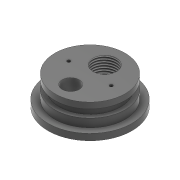
# Autodesk Inventor part: Pieza_sonar
Saved by Autodesk Inventor 2022.3 (Build 263350000, 350)
## iProperties
Created: 2023-07-17
Part Number: Pieza_sonar
Material: Genérico
Document SubType Name: Modeling
Designer: Usuario
Density: 1 g/cm^3
Appearance: Valor por defecto
Author: Usuario
Autodesk Inventor part; units mm, degrees
ref_plane "YZ Plane" through (0, 0, 0) normal (1, 0, 0) x (0, 1, 0)
ref_plane "XZ Plane" through (0, 0, 0) normal (0, 1, 0) x (-1, 0, 0)
sketch "Boceto1" plane through (0, 0, 0) normal (0, 1, 0) x (-1, 0, 0)
  circle A0 centre (0, 0) radius 26
  dimension "d0" = 52
  constraints: 1 centre point, 1 coincident
  measures "d0" diameter of A0
extrude "Extrusión1" add sketch "Boceto1" along normal blind 4
sketch "Boceto2" plane through (0, 4, 0) normal (0, 1, 0) x (1, 0, 0)
  circle A0 centre (0, 0) radius 21.775
  dimension "d3" = 43.55
  constraints: 1 centre point, 1 coincident
  measures "d3" diameter of A0
extrude "Extrusión2" add sketch "Boceto2" along normal blind 13.8
ref_plane "Plano de trabajo1" through (0, 14.2, 0) normal (0, 1, 0) x (1, 0, 0)
sketch "Boceto6" plane through (0, 14.2, 0) normal (0, 1, 0) x (1, 0, 0)
  circle A0 centre (0, 0) radius 21.775
  circle A1 centre (0, 0) radius 18.925
  dimension "d18" = 37.85
  constraints: 2 centre point, 2 coincident
  measures "d18" diameter of A1
extrude "Extrusión6" cut sketch "Boceto6" against normal blind 5
sketch "Boceto7" plane through (0, 0, 0) normal (0, -1, 0) x (1, 0, 0)
  circle A0 centre (0, 0) radius 18.925 projected
  circle A1 centre (0, 0) radius 21.775 projected
  circle A2 centre (0, 0) radius 26 projected
  line L0 (0, 26) -> (0, 20.5)
  line L1 (0, 20.5) -> (0, 3.45)
  arc A3 (8.0792, 17.1138) -> (4.3595, 20.5) centre (0, 11.975) ccw
  line L2 (0, 3.45) -> (4.3595, 3.45)
  line L3 (0, 3.45) -> (-4.3595, 3.45)
  line L4 (0, 20.5) -> (4.3595, 20.5)
  line L5 (0, 20.5) -> (-4.3595, 20.5)
  arc A4 (4.3595, 3.45) -> (8.0792, 17.1138) centre (0, 11.975) ccw
  arc A5 (-4.3595, 3.45) -> (4.3595, 3.45) centre (0, 11.975) ccw
  arc A6 (4.3595, 20.5) -> (-4.3595, 20.5) centre (0, 11.975) ccw
  arc A7 (-4.3595, 20.5) -> (-4.3595, 3.45) centre (0, 11.975) ccw
  dimension "d21" = 5.5
  dimension "d22" = 17.05
  dimension "d23" = 19.15
  constraints: 13 point on circle, 12 end point, 5 centre point, 2 point on line, 2 vertical, 1 horizontal, 1 midpoint, 1 parallel, 1 vertical alignment, 3 other
  measures "d21" distance of L0.start L0.end
  measures "d22" distance of L0.end L1.end
  measures "d23" diameter of A3
extrude "Extrusión7" cut sketch "Boceto7" against normal blind 4.45 contours A4 L2 L1 A0 | A0 L1 L4 A3 | A7 L5 L1 A0 | A0 L1 L3 A7
sketch "Boceto8" plane through (0, 4.45, 0) normal (0, -1, 0) x (1, 0, 0)
  arc A0 (-4.3595, 20.5) -> (-4.3595, 3.45) centre (0, 11.975) ccw projected
  circle A1 centre (0, 11.975) radius 5.275
  point P0 (0, 0)
  dimension "d26" = 10.55
  constraints: 1 centre point, 1 coincident
  measures "d26" diameter of A1
extrude "Extrusión8" cut sketch "Boceto8" against normal blind 15
sketch "Boceto9" plane through (0, 0, 0) normal (0, -1, 0) x (1, 0, 0)
  line L0 (4.3595, 3.45) -> (-4.3595, 3.45) projected
  line L1 (0, 3.45) -> (0, 2.45)
  line L2 (0, 2.45) -> (0, -20.8)
  circle A0 centre (0, -9.175) radius 11.625
  point P0 (0, 0)
  dimension "d29" = 1
  dimension "d30" = 23.25
  constraints: 4 end point, 2 midpoint, 1 point on line, 1 vertical, 1 vertical alignment, 2 other
  measures "d29" distance of L1.start L1.end
  measures "d30" distance of L1.end L2.end
extrude "Extrusión9" cut sketch "Boceto9" against normal blind 4.25
sketch "Boceto10" plane through (0, 4.25, -9.175) normal (0, -1, 0) x (1, 0, 0)
  circle A0 centre (0, 0) radius 7.275
  point P0 (0, 9.175)
  dimension "d33" = 14.55
  constraints: 1 centre point
  measures "d33" diameter of A0
extrude "Extrusión10" cut sketch "Boceto10" against normal up to surface (13.55 mm away)
thread "Rosca2" size "M15x1.5" class "6H" standard "ANSI Metric M Profile" full length
sketch "Boceto11" plane through (0, 17.8, 0) normal (0, 1, 0) x (1, 0, 0)
  line L0 (0, 0) -> (-13.15, 0)
  line L1 (0, 0) -> (13.15, 0)
  circle A0 centre (-13.15, 0) radius 1
  circle A1 centre (13.15, 0) radius 1
  dimension "d38" = 13.15
  dimension "d39" = 13.15
  dimension "d40" = 2
  dimension "d41" = 2
  constraints: 4 end point, 2 centre point, 2 coincident, 2 horizontal
  measures "d38" distance of L0.start L0.end
  measures "d39" distance of L0.start L1.end
  measures "d40" diameter of A0
  measures "d41" diameter of A1
extrude "Extrusión11" cut sketch "Boceto11" against normal blind 5
